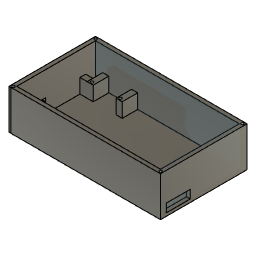
Solar Panel Box (Autodesk Fusion 360 design; units mm, degrees)
Autodesk Fusion 360 part; units mm, degrees
box "BoxPrimitive2" add length 2.6162 width 190.5 height 50.8 placed x (0, -1, 0) y (1, 0, 0) z (0, 0, 1) at (0, 2.54, 0) makes body 1
box "BoxPrimitive3" add length 104.775 width 2.6162 height 50.8 placed x (0, -1, 0) y (1, 0, 0) z (0, 0, 1) at (-2.6162, 0, 0) bodies 1
extrude "Extrude1" add 1 faces at (0, 0.8467, 16.9333) along direction (-1, 0, 0) blind 2.54 on bodies 1 bodies 1
sketch "Sketch4" plane through (0, 0, 0) normal (0, 1, 0) x (-1, 0, 0)
  line L0 (2.54, 50.8) -> (2.54, 0)
  line L1 (2.54, 0) -> (2.6162, 0)
  line L2 (2.6162, 0) -> (2.6162, 50.8)
  line L3 (2.6162, 50.8) -> (2.54, 50.8)
extrude "Extrude2" add sketch "Sketch4" along normal blind 2.54 bodies 1
copy_body "CopyPasteBodies1" bodies 1 makes body 2
move_body "Move1" bodies 2 to x (-1, 0, 0) y (0, -1, 0) z (0, 0, 1) at (190.5, -104.5602, 0)
sketch "Sketch5" plane through (0, 0, 0) normal (-1, 0, 0) x (0, -1, 0)
  line L0 (104.484, 50.8) -> (104.484, 0)
  line L1 (104.484, 0) -> (107.1002, 0)
  line L2 (107.1002, 0) -> (107.1002, 50.8)
  line L3 (107.1002, 50.8) -> (104.484, 50.8)
extrude "Extrude3" add sketch "Sketch5" along normal blind 2.5654 bodies 1 2
extrude "Extrude4" add 1 faces at (-2.5993, -104.775, 16.9333) along direction (0, -1, 0) blind 2.3114 on bodies 1 bodies 1
extrude "Extrude5" add 1 faces at (190.5, 0.9899, 16.9333) along direction (1, 0, 0) blind 2.5654 on bodies 1 bodies 1
extrude "Extrude6" add 1 faces at (193.0993, 0.2148, 16.9333) along direction (0, 1, 0) blind 2.3114 on bodies 1 bodies 1
box "BoxPrimitive4" add length 104.3259 width 190.8753 height 1.905 placed x (0, -1, 0) y (1, 0, 0) z (0, 0, 1) at (0, 0, 0) bodies 1
extrude "Extrude7" add 1 faces at (127.0169, -106.2281, 50.8) along direction (0, 0, 1) blind 1.905 on bodies 1 bodies 1
sketch "Sketch7" plane through (0, -0.0762, 0) normal (0, -1, 0) x (1, 0, 0)
  line L0 (0, 1.905) -> (190.5, 1.905)
  line L1 (190.5, 1.905) -> (190.5, 52.705)
  line L2 (190.5, 52.705) -> (0, 52.705)
  line L3 (0, 52.705) -> (0, 1.905)
sketch "Sketch8" plane through (193.1162, 0, 0) normal (1, 0, 0) x (0, 1, 0)
  line L0 (-107.1002, 0) -> (2.5262, 0)
  line L1 (2.5262, 0) -> (2.5262, 52.705)
  line L2 (2.5262, 52.705) -> (-107.1002, 52.705)
  line L3 (-107.1002, 52.705) -> (-107.1002, 0)
extrude "Extrude8" add 1 faces at (63.5, -104.3259, 0.635) along direction (0, -1, 0) blind 0.4826 on bodies 1 bodies 1
sketch "Sketch9" plane through (190.5, 0, 0) normal (-1, 0, 0) x (0, -1, 0)
  line L0 (0.0762, 1.905) -> (104.484, 1.905)
  line L1 (104.484, 1.905) -> (104.484, 52.705)
  line L2 (104.484, 52.705) -> (0.0762, 52.705)
  line L3 (0.0762, 52.705) -> (0.0762, 1.905)
  line L4 (101.8973, 3.9997) -> (70.1473, 3.9997)
  line L5 (70.1473, 3.9997) -> (70.1473, 15.1342)
  line L6 (70.1473, 15.1342) -> (101.8973, 15.1342)
  line L7 (101.8973, 15.1342) -> (101.8973, 3.9997)
  dimension "d39" = 31.75
  constraint horizontal L4
  constraint vertical L5
  constraint horizontal L6
  constraint vertical L7
  measures "d39" distance of L4.start L4.end
extrude "Extrude9" cut sketch "Sketch9" against normal blind 27.8892 contours L4 L5 L6 L7 bodies 1
extrude "Extrude10" add 1 faces at (127.8382, 2.54, 35.1367) along direction (0, 1, 0) blind 1.905 on bodies 1 bodies 1
extrude "Extrude11" add sketch "Sketch8" along normal blind 1.905 bodies 1
extrude "Extrude12" add 1 faces at (193.0654, 3.8054, 35.1367) along direction (1, 0, 0) blind 1.9558 on bodies 1 bodies 1
extrude "Extrude13" add 1 faces at (63.2968, -107.1002, 35.1367) along direction (0, -1, 0) blind 1.905 on bodies 1 bodies 1
extrude "Extrude14" add 1 faces at (-2.6162, -69.9093, 17.5683) along direction (-1, 0, 0) blind 1.905 on bodies 1 bodies 1
extrude "Extrude15" add 1 faces at (-3.8693, -107.0864, 35.1367) along direction (0, -1, 0) blind 1.905 on bodies 1 bodies 1
sketch "Sketch10" plane through (190.5, 0, 0) normal (-1, 0, 0) x (0, -1, 0)
  line L0 (70.1473, 3.9997) -> (70.1473, 15.1342)
  line L1 (70.1473, 15.1342) -> (101.8973, 15.1342)
  line L2 (101.8973, 15.1342) -> (101.8973, 3.9997)
  line L3 (101.8973, 3.9997) -> (70.1473, 3.9997)
  line L4 (0.0762, 1.905) -> (104.484, 1.905)
  line L5 (104.484, 1.905) -> (104.484, 52.705)
  line L6 (104.484, 52.705) -> (0.0762, 52.705)
  line L7 (0.0762, 52.705) -> (0.0762, 1.905)
extrude "Extrude16" cut sketch "Sketch9" against normal blind 35.941 contours L4 L5 L6 L7 bodies 1
hole "Hole1" at (192.5037, 1.8952, 52.705) direction (0, 0, -1) diameter 4 depth 12.7 tip angle 180 bodies 1
delete_face "DeleteFace1" 1 faces at (194.0033, 3.2186, 48.4717) on bodies 1
extrude "Extrude17" add 1 faces at (195.0212, -26.8461, 14.6682) along direction (1, 0, 0) blind 0.635 on bodies 1 bodies 1
extrude "Extrude18" add 1 faces at (55.5767, 4.445, 30.9033) along direction (0, 1, 0) blind 0.635 on bodies 1 bodies 1
extrude "Extrude19" add 1 faces at (63.5085, -109.0052, 35.1367) along direction (0, -1, 0) blind 0.635 on bodies 1 bodies 1
extrude "Extrude20" add 1 faces at (-4.5212, -32.9438, 35.1367) along direction (-1, 0, 0) blind 0.635 on bodies 1 bodies 1
extrude "Extrude21" add 1 faces at (-3.429, -108.9914, 17.5683) along direction (0, -1, 0) blind 0.635 on bodies 1 bodies 1
hole "Hole2" at (-2.1342, -106.7845, 52.705) direction (0, 0, -1) diameter 3.9878 depth 19.05 tip angle 180 bodies 1
thread "Thread1" "ANSI Unified Screw Threads 0.164(#8) 8-32 UNC 3B" major diameter 4.1656 minor diameter 3.4163 pitch 0.7937 angle 60 resizes the face on face at (-3.9085, -105.8749, 46.355) on bodies 1
hole "Hole3" at (-2.0747, 2.1153, 52.705) direction (0, 0, -1) diameter 3.9878 depth 19.05 tip angle 180 bodies 1
thread "Thread2" "ANSI Unified Screw Threads 0.164(#8) 8-32 UNC 3B" major diameter 4.1656 minor diameter 3.4163 pitch 0.7937 angle 60 resizes the face on face at (-1.8762, 0.1313, 46.355) on bodies 1
hole "Hole4" at (192.8437, -106.6287, 52.705) direction (0, 0, -1) diameter 3.9878 depth 19.05 tip angle 180 bodies 1
thread "Thread3" "ANSI Unified Screw Threads 0.164(#8) 8-32 UNC 3B" major diameter 4.1656 minor diameter 3.4163 pitch 0.7937 angle 60 resizes the face on face at (193.7973, -104.8776, 46.355) on bodies 1
hole "Hole5" at (192.5868, 2.0691, 52.705) direction (0, 0, -1) diameter 3.9878 depth 19.05 tip angle 180 bodies 1
thread "Thread4" "ANSI Unified Screw Threads 0.164(#8) 8-32 UNC 3B" major diameter 4.1656 minor diameter 3.4163 pitch 0.7937 angle 60 resizes the face on face at (193.5404, 3.8202, 46.355) on bodies 1
sketch "Sketch11" plane through (0, 0, 0) normal (1, 0, 0) x (0, 1, 0)
  line L0 (-104.484, 1.905) -> (-0.0762, 1.905)
  line L1 (-0.0762, 1.905) -> (-0.0762, 52.705)
  line L2 (-0.0762, 52.705) -> (-104.484, 52.705)
  line L3 (-104.484, 52.705) -> (-104.484, 1.905)
  line L4 (-75.8115, 20.5042) -> (-66.2865, 20.5042)
  line L5 (-66.2865, 20.5042) -> (-66.2865, 15.7306)
  line L6 (-66.2865, 15.7306) -> (-75.8115, 15.7306)
  line L7 (-75.8115, 15.7306) -> (-75.8115, 20.5042)
  dimension "d81" = 9.525
  constraint horizontal L4
  constraint vertical L5
  constraint horizontal L6
  constraint vertical L7
  measures "d81" distance of L4.start L4.end
extrude "Extrude22" cut sketch "Sketch11" against normal blind 39.7002 contours L4 L5 L6 L7 bodies 1
box "BoxPrimitive5" add length 8.1002 width 8.1026 height 2.54 placed x (0, -1, 0) y (1, 0, 0) z (0, 0, 1) at (12.9167, -25.0896, 1.905) bodies 1
extrude "Extrude23" add 1 faces at (18.3185, -25.0896, 2.7517) along direction (0, 1, 0) blind 12.446 on bodies 1 bodies 1
extrude "Extrude24" cut 1 faces at (18.3185, -33.1898, 2.7517) along direction (0, 1, 0) blind 12.446 on bodies 1 bodies 1
extrude "Extrude25" add 1 faces at (12.9167, -18.0438, 3.5983) along direction (-1, 0, 0) blind 3.4036 on bodies 1 bodies 1
extrude "Extrude26" cut 1 faces at (21.0193, -18.0438, 3.5983) along direction (-1, 0, 0) blind 3.4036 on bodies 1 bodies 1
extrude "Extrude27" add 1 faces at (12.214, -15.3437, 4.445) along direction (0, 0, 1) blind 16.51 on bodies 1 bodies 1
hole "Hole6" at (13.5049, -16.8536, 20.955) direction (0, 0, -1) diameter 3.9878 depth 17.526 tip angle 180 bodies 1
thread "Thread5" "ANSI Unified Screw Threads 0.164(#8) 8-32 UNC 3B" major diameter 4.1656 minor diameter 3.4163 pitch 0.7937 angle 60 resizes the face on face at (13.7034, -18.8376, 15.113) on bodies 1
extrude "Extrude28" add 1 faces at (12.214, -12.6436, 14.605) along direction (0, 1, 0) blind 13.6906 on bodies 1 bodies 1
box "BoxPrimitive6" add length 7.5851 width 10.7758 height 19.0694 placed x (0, 1, 0) y (-1, 0, 0) z (0, 0, 1) at (9.5131, -20.7438, 1.905) bodies 1
box "BoxPrimitive7" add length 7.8411 width 8.1078 height 2.54 placed x (0, 1, 0) y (-1, 0, 0) z (0, 0, 1) at (53.7673, -20.2274, 1.905) bodies 1
extrude "Extrude29" cut 1 faces at (51.0647, -12.3863, 2.7517) along direction (0, -1, 0) blind 0.381 on bodies 1 bodies 1
extrude "Extrude30" add 1 faces at (51.0647, -20.2274, 2.7517) along direction (0, -1, 0) blind 0.381 on bodies 1 bodies 1
extrude "Extrude31" cut 1 faces at (45.6595, -15.381, 2.7517) along direction (1, 0, 0) blind 2.1209 on bodies 1 bodies 1
extrude "Extrude32" add 1 faces at (53.7673, -15.381, 2.7517) along direction (1, 0, 0) blind 2.1209 on bodies 1 bodies 1
extrude "Extrude33" add 1 faces at (50.483, -15.381, 4.445) along direction (0, 0, 1) blind 16.51 on bodies 1 bodies 1
extrude "Extrude34" add 1 faces at (53.1856, -12.7673, 8.255) along direction (0, 1, 0) blind 12.9794 on bodies 1 bodies 1
hole "Hole7" at (50.732, -17.7283, 20.955) direction (0, 0, -1) diameter 3.9878 depth 17.526 tip angle 180 bodies 1
delete_face "DeleteFace2" 1 faces at (15.1241, -17.3976, 15.113) on bodies 1
hole "Hole8" at (14.6021, -17.8526, 20.955) direction (0, 0, -1) diameter 3.9878 depth 17.526 tip angle 180 bodies 1
delete_face "DeleteFace3" 1 faces at (14.8007, -19.8366, 15.113) on bodies 1
hole "Hole9" at (14.5491, -17.8578, 20.955) direction (0, 0, -1) diameter 3.9878 depth 17.526 tip angle 180 bodies 1
delete_face "DeleteFace4" 1 faces at (14.7477, -19.8418, 15.113) on bodies 1
hole "Hole10" at (13.8292, -17.8152, 20.955) direction (0, 0, -1) diameter 3.9878 depth 17.526 tip angle 180 bodies 1
delete_face "DeleteFace5" 1 faces at (14.0278, -19.7992, 15.113) on bodies 1
hole "Hole11" at (13.1993, -17.8781, 20.955) direction (0, 0, -1) diameter 3.9878 depth 17.526 tip angle 180 bodies 1
thread "Thread6" "ANSI Unified Screw Threads 0.164(#8) 8-32 UNC 3B" major diameter 4.1656 minor diameter 3.4163 pitch 0.7937 angle 60 resizes the face on face at (13.3978, -19.8621, 15.113) on bodies 1
thread "Thread7" "ANSI Unified Screw Threads 0.164(#8) 8-32 UNC 3B" major diameter 4.1656 minor diameter 3.4163 pitch 0.7937 angle 60 resizes the face on face at (50.337, -15.774, 15.113) on bodies 1
